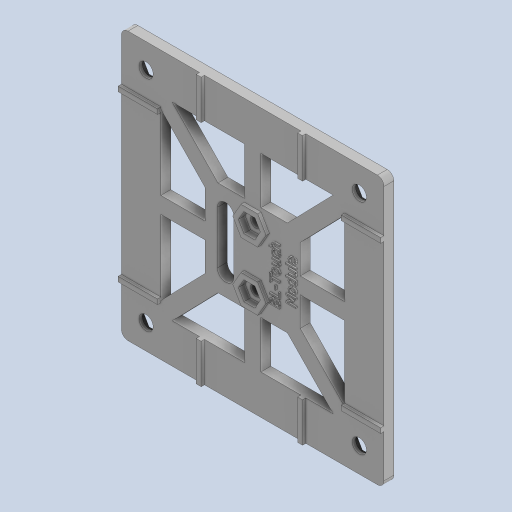
# Autodesk Inventor part: BLTouch-LevelingPlate
Saved by Autodesk Inventor 2023.2 (Build 272271000, 271)
## iProperties
Created: 2024-02-15
Part Number: BLTouch-LevelingPlate
Material: Generisch
Document SubType Name: Modeling
Designer: Nils Bade
Density: 1 g/cm^3
Appearance: PLA Druck IHF
Description: Dummy
Auf Bestellliste: True
Author: Nils Bade
Autodesk Inventor part; units mm, degrees
ref_plane "YZ Plane" through (0, 0, 0) normal (1, 0, 0) x (0, 1, 0)
ref_plane "XZ Plane" through (0, 0, 0) normal (0, 1, 0) x (-1, 0, 0)
ref_plane "XY Plane" through (0, 0, 0) normal (0, 0, 1) x (1, 0, 0)
sketch "S-Basis" plane through (0, 0, 0) normal (0, 0, 1) x (1, 0, 0)
  line L0 (0, 57.19) -> (0, -57.19) construction
  line L1 (-56, 0) -> (56, 0) construction
  line L2 (-40, 40.85) -> (40, 40.85)
  line L3 (40, 40.85) -> (40, -40.85)
  line L4 (40, -40.85) -> (-40, -40.85)
  line L5 (-40, -40.85) -> (-40, 40.85)
  line L6 (-40, 40.85) -> (40, -40.85) construction
  line L7 (40, 40.85) -> (-40, -40.85) construction
  line L8 (-40, 33.35) -> (40, 33.35) construction
  circle A0 centre (0, 33.35) radius 2.5 construction
  circle A1 centre (-32.5, 33.35) radius 2.15
  circle A2 centre (32.5, 33.35) radius 2.15
  circle A3 centre (-32.5, -33.35) radius 2.15
  circle A4 centre (32.5, -33.35) radius 2.15
  line L9 (-3.5, 40.85) -> (3.5, 40.85)
  line L10 (7.5, 31.85) -> (5, 31.85)
  line L11 (5, 31.85) -> (5, 37.85)
  line L12 (5, 37.85) -> (7.5, 37.85)
  line L13 (7.5, 37.85) -> (7.5, 31.85)
  line L14 (-7.5, 31.85) -> (-5, 31.85)
  line L15 (-5, 31.85) -> (-5, 37.85)
  line L16 (-5, 37.85) -> (-7.5, 37.85)
  line L17 (-7.5, 37.85) -> (-7.5, 31.85)
  point P0 (0, 40.85)
  point P1 (0, 0)
  point P2 (0, 0)
  dimension "d0" = 81.7
  dimension "d1" = 80
  dimension "d4" = 7.5
  dimension "d7" = 4.3
  dimension "d8" = 32.5
  dimension "d9" = 4.3
  dimension "d10" = 32.5
  dimension "d11" = 7.5
  dimension "d60" = 6
  dimension "d61" = 2.5
  dimension "d62" = 5
  dimension "d63" = 3
  constraints: 32 end point, 6 midpoint, 6 symmetric about line, 5 centre point, 5 point on line, 4 parallel, 3 horizontal, 3 perpendicular, 2 other
  measures "d0" distance of L2.end L3.end
  measures "d1" distance of L2.start L2.end
  measures "d4" distance between parallel lines of L8 L2
  measures "d7" diameter of A1
  measures "d8" distance from line of L0 A1.centre
  measures "d9" diameter of A3
  measures "d10" distance from line of L0 A3.centre
  measures "d11" distance from line of L4 A3.centre
  measures "d60" distance of L12.end L10.start
  measures "d61" distance between parallel lines of L13 L11
  measures "d62" distance between parallel lines of L0 L11
  measures "d63" distance between parallel lines of L12 L2
extrude "Ex-Base1" add sketch "S-Basis" against normal blind 3 contours L2 L3 L4 L5 | L10 L11 L12 L13 | L17 L16 L15 L14
fillet "Rundung-2mm" radius 2 4 edges at (40, -40.85, -1.5) (-40, -40.85, -1.5) (40, 40.85, -1.5) (-40, 40.85, -1.5)
sketch "S-BLTouch-Mount" plane through (0, 0, 0) normal (0, 0, 1) x (1, 0, 0)
  line L0 (0, 9) -> (0, -9) construction
  line L1 (-4.4389, 9) -> (-4.4389, -9) construction
  line L2 (4.4389, -9) -> (4.4389, 9) construction
  arc A0 (4.4389, 9) -> (-4.4389, 9) centre (0, 9) ccw construction
  arc A1 (-4.4389, -9) -> (4.4389, -9) centre (0, -9) ccw construction
  circle A2 centre (0, -9) radius 1.65
  line L3 (0, 57.19) -> (0, -57.19) construction
  line L4 (-56, 0) -> (56, 0) construction
  line L5 (-1.6743, -6.1) -> (1.6743, -6.1)
  line L6 (1.6743, -6.1) -> (3.3486, -9)
  line L7 (3.3486, -9) -> (1.6743, -11.9)
  line L8 (1.6743, -11.9) -> (-1.6743, -11.9)
  line L9 (-1.6743, -11.9) -> (-3.3486, -9)
  line L10 (-3.3486, -9) -> (-1.6743, -6.1)
  circle A3 centre (0, 0) radius 3
  line L11 (-8.25, 8) -> (-8.25, -8) construction
  line L12 (-10.75, 8) -> (-10.75, -8)
  line L13 (-5.75, -8) -> (-5.75, 8)
  arc A4 (-5.75, 8) -> (-10.75, 8) centre (-8.25, 8) ccw
  arc A5 (-10.75, -8) -> (-5.75, -8) centre (-8.25, -8) ccw
  circle A6 centre (0, 9) radius 1.65
  line L14 (-1.6743, 6.1) -> (1.6743, 6.1)
  line L15 (1.6743, 6.1) -> (3.3486, 9)
  line L16 (3.3486, 9) -> (1.6743, 11.9)
  line L17 (1.6743, 11.9) -> (-1.6743, 11.9)
  line L18 (-1.6743, 11.9) -> (-3.3486, 9)
  line L19 (-3.3486, 9) -> (-1.6743, 6.1)
  line L20 (-5.0807, -9) -> (-2.5403, -13.4)
  line L21 (-2.5403, -13.4) -> (2.5403, -13.4)
  line L22 (2.5403, -13.4) -> (5.0807, -9)
  line L23 (5.0807, -9) -> (2.5403, -4.6)
  line L24 (2.5403, -4.6) -> (-2.5403, -4.6)
  line L25 (-2.5403, -4.6) -> (-5.0807, -9)
  line L26 (-2.5403, 4.6) -> (2.5403, 4.6)
  line L27 (2.5403, 4.6) -> (5.0807, 9)
  line L28 (5.0807, 9) -> (2.5403, 13.4)
  line L29 (2.5403, 13.4) -> (-2.5403, 13.4)
  line L30 (-2.5403, 13.4) -> (-5.0807, 9)
  line L31 (-5.0807, 9) -> (-2.5403, 4.6)
  line L32 (-14.5, -14.5) -> (14.5, -14.5)
  line L33 (14.5, -14.5) -> (14.5, 14.5)
  line L34 (14.5, 14.5) -> (-14.5, 14.5)
  line L35 (-14.5, 14.5) -> (-14.5, -14.5)
  line L36 (-14.5, -14.5) -> (14.5, 14.5) construction
  line L37 (14.5, -14.5) -> (-14.5, 14.5) construction
  line L38 (28, -28.85) -> (-28, -28.85)
  line L39 (-28, -28.85) -> (-28, 28.85)
  line L40 (-28, 28.85) -> (28, 28.85)
  line L41 (28, 28.85) -> (28, -28.85)
  line L42 (28, -28.85) -> (-28, 28.85) construction
  line L43 (-28, -28.85) -> (28, 28.85) construction
  line L44 (40, -38.85) -> (40, 38.85) projected
  line L45 (-40, 38.85) -> (-40, -38.85) projected
  line L46 (-38, -40.85) -> (38, -40.85) projected
  line L47 (2.5, -28.85) -> (2.5, -14.5)
  line L48 (10.589, -14.5) -> (24.5162, -28.85)
  line L49 (14.5, -11.3506) -> (28, -25.2604)
  line L50 (14.5, -2.5) -> (28, -2.5)
  line L51 (2.5, 28.85) -> (2.5, 14.5)
  line L52 (10.589, 14.5) -> (24.5162, 28.85)
  line L53 (14.5, 11.3506) -> (28, 25.2604)
  line L54 (14.5, 2.5) -> (28, 2.5)
  line L55 (-2.5, -28.85) -> (-2.5, -14.5)
  line L56 (-10.589, -14.5) -> (-24.5162, -28.85)
  line L57 (-14.5, -11.3506) -> (-28, -25.2604)
  line L58 (-14.5, -2.5) -> (-28, -2.5)
  line L59 (-2.5, 28.85) -> (-2.5, 14.5)
  line L60 (-10.589, 14.5) -> (-24.5162, 28.85)
  line L61 (-14.5, 11.3506) -> (-28, 25.2604)
  line L62 (-14.5, 2.5) -> (-28, 2.5)
  line L63 (5.3885, -14.3851) -> (5.3885, 14.3851) construction
  line L64 (5.3885, 14.3851) -> (13.9659, 14.3851) construction
  line L65 (13.9659, 14.3851) -> (13.9659, -14.3851) construction
  line L66 (13.9659, -14.3851) -> (5.3885, -14.3851) construction
  spline S0 degree 2 poles (7.6363, -6.9815) (7.8635, -6.9815) (8.2118, -7.1544) (8.3254, -7.2977) knots 0 0 0 1 2 2 2
  spline S1 degree 2 poles (8.3254, -7.2977) (8.4588, -7.4706) (8.5724, -7.8633) (8.5724, -8.1745) knots 0 0 0 1 2 2 2
  line L67 (8.5724, -8.1745) -> (8.5724, -9.0489)
  line L68 (8.5724, -9.0489) -> (5.5244, -9.0489)
  line L69 (5.5244, -9.0489) -> (5.5244, -8.2412)
  spline S2 degree 2 poles (5.5244, -8.2412) (5.5244, -7.9152) (5.5664, -7.5891) (5.6479, -7.4409) knots 0 0 0 1 2 2 2
  spline S3 degree 2 poles (5.6479, -7.4409) (5.7343, -7.2754) (6.0184, -7.1248) (6.2111, -7.1248) knots 0 0 0 1 2 2 2
  spline S4 degree 2 poles (6.2111, -7.1248) (6.4259, -7.1248) (6.7668, -7.352) (6.8631, -7.5521) knots 0 0 0 1 2 2 2
  line L70 (6.8631, -7.5521) -> (6.878, -7.5521)
  spline S5 degree 2 poles (6.878, -7.5521) (6.9521, -7.2804) (7.3448, -6.9815) (7.6363, -6.9815) knots 0 0 0 1 2 2 2
  spline S6 degree 2 poles (7.6535, -7.4039) (7.4806, -7.4039) (7.2583, -7.5027) (7.1793, -7.6509) knots 0 0 0 1 2 2 2
  spline S7 degree 2 poles (7.1793, -7.6509) (7.1299, -7.7472) (7.1003, -7.9744) (7.1003, -8.1844) knots 0 0 0 1 2 2 2
  line L71 (7.1003, -8.1844) -> (7.1003, -8.6438)
  line L72 (7.1003, -8.6438) -> (8.2266, -8.6438)
  line L73 (8.2266, -8.6438) -> (8.2266, -8.3153)
  spline S8 degree 2 poles (8.2266, -8.3153) (8.2266, -8.0485) (8.1772, -7.7423) (8.0981, -7.6237) knots 0 0 0 1 2 2 2
  spline S9 degree 2 poles (8.0981, -7.6237) (8.0166, -7.5101) (7.8141, -7.4039) (7.6535, -7.4039) knots 0 0 0 1 2 2 2
  spline S10 degree 2 poles (6.2679, -7.5471) (6.1592, -7.5471) (5.9962, -7.6212) (5.9492, -7.7027) knots 0 0 0 1 2 2 2
  spline S11 degree 2 poles (5.9492, -7.7027) (5.8949, -7.8015) (5.8702, -8.0411) (5.8702, -8.256) knots 0 0 0 1 2 2 2
  line L74 (5.8702, -8.256) -> (5.8702, -8.6438)
  line L75 (5.8702, -8.6438) -> (6.7619, -8.6438)
  line L76 (6.7619, -8.6438) -> (6.7619, -8.1844)
  spline S12 degree 2 poles (6.7619, -8.1844) (6.7619, -7.9942) (6.7223, -7.8139) (6.6606, -7.7176) knots 0 0 0 1 2 2 2
  spline S13 degree 2 poles (6.6606, -7.7176) (6.6013, -7.6237) (6.4111, -7.5471) (6.2679, -7.5471) knots 0 0 0 1 2 2 2
  line L77 (8.5724, -4.8128) -> (8.5724, -6.5789)
  line L78 (8.5724, -6.5789) -> (5.5244, -6.5789)
  line L79 (5.5244, -6.5789) -> (5.5244, -6.1738)
  line L80 (5.5244, -6.1738) -> (8.2118, -6.1738)
  line L81 (8.2118, -6.1738) -> (8.2118, -4.8128)
  line L82 (8.2118, -4.8128) -> (8.5724, -4.8128)
  line L83 (7.4238, -3.4642) -> (7.4238, -4.6177)
  line L84 (7.4238, -4.6177) -> (7.0533, -4.6177)
  line L85 (7.0533, -4.6177) -> (7.0533, -3.4642)
  line L86 (7.0533, -3.4642) -> (7.4238, -3.4642)
  line L87 (8.5724, -2.2613) -> (5.885, -2.2613)
  line L88 (5.885, -2.2613) -> (5.885, -3.2839)
  line L89 (5.885, -3.2839) -> (5.5244, -3.2839)
  line L90 (5.5244, -3.2839) -> (5.5244, -0.8336)
  line L91 (5.5244, -0.8336) -> (5.885, -0.8336)
  line L92 (5.885, -0.8336) -> (5.885, -1.8562)
  line L93 (5.885, -1.8562) -> (8.5724, -1.8562)
  line L94 (8.5724, -1.8562) -> (8.5724, -2.2613)
  spline S14 degree 2 poles (7.4288, 1.3252) (8.0068, 1.3252) (8.6366, 0.7694) (8.6366, 0.305) knots 0 0 0 1 2 2 2
  spline S15 degree 2 poles (8.6366, 0.305) (8.6366, -0.1717) (7.987, -0.7175) (7.4288, -0.7175) knots 0 0 0 1 2 2 2
  spline S16 degree 2 poles (7.4288, -0.7175) (6.8557, -0.7175) (6.2209, -0.1544) (6.2209, 0.305) knots 0 0 0 1 2 2 2
  spline S17 degree 2 poles (6.2209, 0.305) (6.2209, 0.7694) (6.8533, 1.3252) (7.4288, 1.3252) knots 0 0 0 1 2 2 2
  spline S18 degree 2 poles (7.4288, 0.9275) (6.9842, 0.9275) (6.5519, 0.6039) (6.5519, 0.305) knots 0 0 0 1 2 2 2
  spline S19 degree 2 poles (6.5519, 0.305) (6.5519, 0.0062) (6.9842, -0.3199) (7.4288, -0.3199) knots 0 0 0 1 2 2 2
  spline S20 degree 2 poles (7.4288, -0.3199) (7.861, -0.3199) (8.3056, 0.0062) (8.3056, 0.305) knots 0 0 0 1 2 2 2
  spline S21 degree 2 poles (8.3056, 0.305) (8.3056, 0.6014) (7.8684, 0.9275) (7.4288, 0.9275) knots 0 0 0 1 2 2 2
  line L95 (8.5724, 3.4988) -> (8.5724, 3.1135)
  line L96 (8.5724, 3.1135) -> (8.3204, 3.1135)
  spline S22 degree 2 poles (8.3204, 3.1135) (8.4761, 2.9356) (8.6366, 2.617) (8.6366, 2.4194) knots 0 0 0 1 2 2 2
  spline S23 degree 2 poles (8.6366, 2.4194) (8.6366, 2.2712) (8.5378, 2.0069) (8.4316, 1.9106) knots 0 0 0 1 2 2 2
  spline S24 degree 2 poles (8.4316, 1.9106) (8.3254, 1.8118) (8.0018, 1.7031) (7.7696, 1.7031) knots 0 0 0 1 2 2 2
  line L97 (7.7696, 1.7031) -> (6.2852, 1.7031)
  line L98 (6.2852, 1.7031) -> (6.2852, 2.0884)
  line L99 (6.2852, 2.0884) -> (7.5893, 2.0884)
  spline S25 degree 2 poles (7.5893, 2.0884) (7.7721, 2.0884) (8.0117, 2.1156) (8.1006, 2.1625) knots 0 0 0 1 2 2 2
  spline S26 degree 2 poles (8.1006, 2.1625) (8.1895, 2.2094) (8.271, 2.37) (8.271, 2.5207) knots 0 0 0 1 2 2 2
  spline S27 degree 2 poles (8.271, 2.5207) (8.271, 2.6614) (8.1105, 2.9801) (7.9944, 3.1135) knots 0 0 0 1 2 2 2
  line L100 (7.9944, 3.1135) -> (6.2852, 3.1135)
  line L101 (6.2852, 3.1135) -> (6.2852, 3.4988)
  line L102 (6.2852, 3.4988) -> (8.5724, 3.4988)
  spline S28 degree 2 poles (8.6243, 4.966) (8.6243, 4.7288) (8.4785, 4.3361) (8.3303, 4.1953) knots 0 0 0 1 2 2 2
  spline S29 degree 2 poles (8.3303, 4.1953) (8.1846, 4.0545) (7.7351, 3.8989) (7.4337, 3.8989) knots 0 0 0 1 2 2 2
  spline S30 degree 2 poles (7.4337, 3.8989) (7.1324, 3.8989) (6.6927, 4.0595) (6.5445, 4.1953) knots 0 0 0 1 2 2 2
  spline S31 degree 2 poles (6.5445, 4.1953) (6.3938, 4.3312) (6.2333, 4.7338) (6.2333, 4.966) knots 0 0 0 1 2 2 2
  spline S32 degree 2 poles (6.2333, 4.966) (6.2333, 5.1537) (6.3395, 5.5044) (6.4087, 5.6403) knots 0 0 0 1 2 2 2
  line L103 (6.4087, 5.6403) -> (6.8409, 5.6403)
  line L104 (6.8409, 5.6403) -> (6.8409, 5.6181)
  spline S33 degree 2 poles (6.8409, 5.6181) (6.8063, 5.5761) (6.7174, 5.4476) (6.6705, 5.3562) knots 0 0 0 1 2 2 2
  spline S34 degree 2 poles (6.6705, 5.3562) (6.631, 5.2747) (6.5692, 5.0574) (6.5692, 4.9586) knots 0 0 0 1 2 2 2
  spline S35 degree 2 poles (6.5692, 4.9586) (6.5692, 4.6597) (7.0212, 4.2966) (7.4337, 4.2966) knots 0 0 0 1 2 2 2
  spline S36 degree 2 poles (7.4337, 4.2966) (7.8363, 4.2966) (8.2883, 4.6473) (8.2883, 4.9586) knots 0 0 0 1 2 2 2
  spline S37 degree 2 poles (8.2883, 4.9586) (8.2883, 5.1463) (8.1327, 5.4871) (8.0117, 5.6181) knots 0 0 0 1 2 2 2
  line L105 (8.0117, 5.6181) -> (8.0117, 5.6403)
  line L106 (8.0117, 5.6403) -> (8.4439, 5.6403)
  spline S38 degree 2 poles (8.4439, 5.6403) (8.4711, 5.5835) (8.5477, 5.4106) (8.565, 5.3414) knots 0 0 0 1 2 2 2
  spline S39 degree 2 poles (8.565, 5.3414) (8.5946, 5.2426) (8.6243, 5.087) (8.6243, 4.966) knots 0 0 0 1 2 2 2
  line L107 (8.5724, 7.7867) -> (8.5724, 7.4014)
  line L108 (8.5724, 7.4014) -> (7.2682, 7.4014)
  spline S40 degree 2 poles (7.2682, 7.4014) (7.1101, 7.4014) (6.8384, 7.3718) (6.7569, 7.3273) knots 0 0 0 1 2 2 2
  spline S41 degree 2 poles (6.7569, 7.3273) (6.6705, 7.2804) (6.5865, 7.1124) (6.5865, 6.9692) knots 0 0 0 1 2 2 2
  spline S42 degree 2 poles (6.5865, 6.9692) (6.5865, 6.8259) (6.7396, 6.5221) (6.8631, 6.3763) knots 0 0 0 1 2 2 2
  line L109 (6.8631, 6.3763) -> (8.5724, 6.3763)
  line L110 (8.5724, 6.3763) -> (8.5724, 5.991)
  line L111 (8.5724, 5.991) -> (5.3885, 5.991)
  line L112 (5.3885, 5.991) -> (5.3885, 6.3763)
  line L113 (5.3885, 6.3763) -> (6.5396, 6.3763)
  spline S43 degree 2 poles (6.5396, 6.3763) (6.384, 6.5492) (6.2209, 6.8827) (6.2209, 7.0704) knots 0 0 0 1 2 2 2
  spline S44 degree 2 poles (6.2209, 7.0704) (6.2209, 7.4063) (6.6655, 7.7867) (7.0879, 7.7867) knots 0 0 0 1 2 2 2
  line L114 (7.0879, 7.7867) -> (8.5724, 7.7867)
  line L115 (13.5908, -3.7396) -> (13.5908, -4.1447)
  line L116 (13.5908, -4.1447) -> (10.9652, -4.1447)
  line L117 (10.9652, -4.1447) -> (12.751, -4.94)
  line L118 (12.751, -4.94) -> (12.751, -5.187)
  line L119 (12.751, -5.187) -> (10.9652, -5.975)
  line L120 (10.9652, -5.975) -> (13.5908, -5.975)
  line L121 (13.5908, -5.975) -> (13.5908, -6.3529)
  line L122 (13.5908, -6.3529) -> (10.5428, -6.3529)
  line L123 (10.5428, -6.3529) -> (10.5428, -5.7996)
  line L124 (10.5428, -5.7996) -> (12.2397, -5.0388)
  line L125 (12.2397, -5.0388) -> (10.5428, -4.3028)
  line L126 (10.5428, -4.3028) -> (10.5428, -3.7396)
  line L127 (10.5428, -3.7396) -> (13.5908, -3.7396)
  spline S45 degree 2 poles (12.4472, -1.2721) (13.0252, -1.2721) (13.6551, -1.8278) (13.6551, -2.2922) knots 0 0 0 1 2 2 2
  spline S46 degree 2 poles (13.6551, -2.2922) (13.6551, -2.7689) (13.0054, -3.3148) (12.4472, -3.3148) knots 0 0 0 1 2 2 2
  spline S47 degree 2 poles (12.4472, -3.3148) (11.8742, -3.3148) (11.2394, -2.7516) (11.2394, -2.2922) knots 0 0 0 1 2 2 2
  spline S48 degree 2 poles (11.2394, -2.2922) (11.2394, -1.8278) (11.8717, -1.2721) (12.4472, -1.2721) knots 0 0 0 1 2 2 2
  spline S49 degree 2 poles (12.4472, -1.6697) (12.0026, -1.6697) (11.5704, -1.9933) (11.5704, -2.2922) knots 0 0 0 1 2 2 2
  spline S50 degree 2 poles (11.5704, -2.2922) (11.5704, -2.591) (12.0026, -2.9171) (12.4472, -2.9171) knots 0 0 0 1 2 2 2
  spline S51 degree 2 poles (12.4472, -2.9171) (12.8795, -2.9171) (13.3241, -2.591) (13.3241, -2.2922) knots 0 0 0 1 2 2 2
  spline S52 degree 2 poles (13.3241, -2.2922) (13.3241, -1.9958) (12.8869, -1.6697) (12.4472, -1.6697) knots 0 0 0 1 2 2 2
  line L128 (13.5908, 0.8818) -> (13.5908, 0.4965)
  line L129 (13.5908, 0.4965) -> (13.3587, 0.4965)
  spline S53 degree 2 poles (13.3587, 0.4965) (13.4328, 0.4076) (13.5316, 0.2766) (13.5735, 0.1877) knots 0 0 0 1 2 2 2
  spline S54 degree 2 poles (13.5735, 0.1877) (13.6131, 0.1062) (13.6551, -0.0692) (13.6551, -0.1853) knots 0 0 0 1 2 2 2
  spline S55 degree 2 poles (13.6551, -0.1853) (13.6551, -0.373) (13.4994, -0.6891) (13.3488, -0.8003) knots 0 0 0 1 2 2 2
  spline S56 degree 2 poles (13.3488, -0.8003) (13.1981, -0.9114) (12.7535, -1.0349) (12.4645, -1.0349) knots 0 0 0 1 2 2 2
  spline S57 degree 2 poles (12.4645, -1.0349) (12.1632, -1.0349) (11.7235, -0.8793) (11.558, -0.7435) knots 0 0 0 1 2 2 2
  spline S58 degree 2 poles (11.558, -0.7435) (11.4098, -0.6175) (11.2394, -0.2643) (11.2394, -0.0692) knots 0 0 0 1 2 2 2
  spline S59 degree 2 poles (11.2394, -0.0692) (11.2394, 0.1013) (11.316, 0.3557) (11.395, 0.4965) knots 0 0 0 1 2 2 2
  line L130 (11.395, 0.4965) -> (10.407, 0.4965)
  line L131 (10.407, 0.4965) -> (10.407, 0.8818)
  line L132 (10.407, 0.8818) -> (13.5908, 0.8818)
  line L133 (13.0351, 0.4965) -> (11.7136, 0.4965)
  spline S60 degree 2 poles (11.7136, 0.4965) (11.6445, 0.3532) (11.5926, 0.126) (11.5926, -0.0049) knots 0 0 0 1 2 2 2
  spline S61 degree 2 poles (11.5926, -0.0049) (11.5926, -0.3013) (12.0372, -0.6373) (12.4571, -0.6373) knots 0 0 0 1 2 2 2
  spline S62 degree 2 poles (12.4571, -0.6373) (12.8622, -0.6373) (13.2895, -0.3804) (13.2895, -0.0963) knots 0 0 0 1 2 2 2
  spline S63 degree 2 poles (13.2895, -0.0963) (13.2895, 0.0543) (13.1512, 0.3606) (13.0351, 0.4965) knots 0 0 0 1 2 2 2
  line L134 (13.5908, 3.2184) -> (13.5908, 2.8331)
  line L135 (13.5908, 2.8331) -> (13.3389, 2.8331)
  spline S64 degree 2 poles (13.3389, 2.8331) (13.4945, 2.6553) (13.6551, 2.3366) (13.6551, 2.139) knots 0 0 0 1 2 2 2
  spline S65 degree 2 poles (13.6551, 2.139) (13.6551, 1.9908) (13.5563, 1.7265) (13.45, 1.6302) knots 0 0 0 1 2 2 2
  spline S66 degree 2 poles (13.45, 1.6302) (13.3438, 1.5314) (13.0203, 1.4227) (12.7881, 1.4227) knots 0 0 0 1 2 2 2
  line L136 (12.7881, 1.4227) -> (11.3036, 1.4227)
  line L137 (11.3036, 1.4227) -> (11.3036, 1.8081)
  line L138 (11.3036, 1.8081) -> (12.6078, 1.8081)
  spline S67 degree 2 poles (12.6078, 1.8081) (12.7906, 1.8081) (13.0301, 1.8352) (13.1191, 1.8822) knots 0 0 0 1 2 2 2
  spline S68 degree 2 poles (13.1191, 1.8822) (13.208, 1.9291) (13.2895, 2.0896) (13.2895, 2.2403) knots 0 0 0 1 2 2 2
  spline S69 degree 2 poles (13.2895, 2.2403) (13.2895, 2.3811) (13.1289, 2.6997) (13.0129, 2.8331) knots 0 0 0 1 2 2 2
  line L139 (13.0129, 2.8331) -> (11.3036, 2.8331)
  line L140 (11.3036, 2.8331) -> (11.3036, 3.2184)
  line L141 (11.3036, 3.2184) -> (13.5908, 3.2184)
  line L142 (13.5908, 4.1694) -> (13.5908, 3.7841)
  line L143 (13.5908, 3.7841) -> (10.407, 3.7841)
  line L144 (10.407, 3.7841) -> (10.407, 4.1694)
  line L145 (10.407, 4.1694) -> (13.5908, 4.1694)
  spline S70 degree 2 poles (13.6427, 5.728) (13.6427, 5.1796) (13.0277, 4.5769) (12.4596, 4.5769) knots 0 0 0 1 2 2 2
  spline S71 degree 2 poles (12.4596, 4.5769) (11.9013, 4.5769) (11.2394, 5.1623) (11.2394, 5.6341) knots 0 0 0 1 2 2 2
  spline S72 degree 2 poles (11.2394, 5.6341) (11.2394, 5.8465) (11.3629, 6.175) (11.4938, 6.2961) knots 0 0 0 1 2 2 2
  spline S73 degree 2 poles (11.4938, 6.2961) (11.6247, 6.4196) (12.0026, 6.5505) (12.2768, 6.5505) knots 0 0 0 1 2 2 2
  line L146 (12.2768, 6.5505) -> (12.4867, 6.5505)
  line L147 (12.4867, 6.5505) -> (12.4867, 4.9672)
  spline S74 degree 2 poles (12.4867, 4.9672) (12.8844, 4.9672) (13.3068, 5.3673) (13.3068, 5.723) knots 0 0 0 1 2 2 2
  spline S75 degree 2 poles (13.3068, 5.723) (13.3068, 5.849) (13.25, 6.0935) (13.2055, 6.1923) knots 0 0 0 1 2 2 2
  spline S76 degree 2 poles (13.2055, 6.1923) (13.1561, 6.2961) (13.0697, 6.4393) (13.0301, 6.4863) knots 0 0 0 1 2 2 2
  line L148 (13.0301, 6.4863) -> (13.0301, 6.5085)
  line L149 (13.0301, 6.5085) -> (13.45, 6.5085)
  spline S77 degree 2 poles (13.45, 6.5085) (13.4772, 6.4418) (13.5563, 6.2393) (13.5785, 6.1602) knots 0 0 0 1 2 2 2
  spline S78 degree 2 poles (13.5785, 6.1602) (13.6106, 6.0491) (13.6427, 5.8663) (13.6427, 5.728) knots 0 0 0 1 2 2 2
  spline S79 degree 2 poles (12.1928, 6.175) (12.0372, 6.1701) (11.81, 6.1059) (11.7334, 6.0441) knots 0 0 0 1 2 2 2
  spline S80 degree 2 poles (11.7334, 6.0441) (11.6469, 5.9774) (11.5555, 5.7675) (11.5555, 5.6119) knots 0 0 0 1 2 2 2
  spline S81 degree 2 poles (11.5555, 5.6119) (11.5555, 5.4587) (11.6469, 5.2438) (11.7359, 5.1549) knots 0 0 0 1 2 2 2
  spline S82 degree 2 poles (11.7359, 5.1549) (11.8272, 5.0685) (12.0471, 4.9796) (12.1928, 4.9672) knots 0 0 0 1 2 2 2
  line L150 (12.1928, 4.9672) -> (12.1928, 6.175)
  point P0 (-8.25, 0)
  point P1 (5.3885, 0)
  dimension "d26" = 18
  dimension "d27" = 3.3
  dimension "d28" = 5.8
  dimension "d29" = 6
  dimension "d30" = 5.75
  dimension "d31" = 5
  dimension "d32" = 16
  dimension "d39" = 1.5
  dimension "d40" = 1.5
  dimension "d43" = 29
  dimension "d44" = 29
  dimension "d45" = 12
  dimension "d46" = 12
  dimension "d47" = 2.5
  dimension "d48" = 5
  dimension "d49" = 2.5
  constraints: 120 end point, 32 symmetric about line, 10 point on line, 8 point on circle, 8 tangent, 7 centre point, 7 midpoint, 7 parallel, 5 coincident, 5 perpendicular, 3 horizontal, 1 vertical, 27 other
  measures "d26" distance of L0.start L0.end
  measures "d27" diameter of A2
  measures "d28" distance between parallel lines of L8 L5
  measures "d29" diameter of A3
  measures "d30" distance between parallel lines of L13 L3
  measures "d31" distance between parallel lines of L13 L12
  measures "d32" distance of L12.start L12.end
  measures "d39" distance between parallel lines of L9 L20
  measures "d40" distance between parallel lines of L19 L31
  measures "d43" distance of L34.end L33.end
  measures "d44" distance of L33.end L32.end
  measures "d45" distance between parallel lines of L38 L46
  measures "d46" distance between parallel lines of L45 L39
  measures "d47" distance between parallel lines of L4 L50
  measures "d48" distance between parallel lines of L49 L48
  measures "d49" distance between parallel lines of L3 L47
extrude "Ex-BLTouch-Mount1" cut sketch "S-BLTouch-Mount" against normal blind 10 contours A2 | A4 L13 A5 L12 | A6
extrude "Ex-BLTouch-Mount2" cut sketch "S-BLTouch-Mount" along normal blind 1 from surface at -3 contours A3
extrude "Ex-BLTouch-Mount3" cut sketch "S-BLTouch-Mount" against normal blind 1 contours L5 L6 L7 L8 L9 L10 | L19 L18 L17 L16 L15 L14
extrude "Ex-BLTouch-Mount4" add sketch "S-BLTouch-Mount" along normal blind 1 contours L25 L24 L23 L22 L21 L20 | L31 L30 L29 L28 L27 L26
extrude "Ex-LightWeightBABY" cut sketch "S-BLTouch-Mount" against normal blind 3 contours L32 L55 L38 L56 | L57 L39 L58 L35 | L32 L48 L38 L47 | L62 L39 L61 L35 | L33 L50 L41 L49 | L60 L40 L59 L34 | L33 L53 L41 L54 | L51 L40 L52 L34
extrude "Ex-Beschriftung" add sketch "S-BLTouch-Mount" along normal blind 0.5 contours S0 S1 L67 L68 L69 S2 S3 S4 L70 S5 | L77 L78 L79 L80 L81 L82 | L83 L84 L85 L86 | L87 L88 L89 L90 L91 L92 L93 L94 | S14 S15 S16 S17 | L95 L96 S22 S23 S24 L97 L98 L99 S25 S26 S27 L100 L101 L102 | S28 S29 S30 S31 S32 L103 L104 S33 S34 S35 S36 S37 L105 L106 S38 S39 | L107 L108 S40 S41 S42 L109 L110 L111 L112 L113 S43 S44 L114 | L115 L116 L117 L118 L119 L120 L121 L122 L123 L124 L125 L126 L127 | S45 S46 S47 S48 | L128 L129 S53 S54 S55 S56 S57 S58 S59 L130 L131 L132 | L134 L135 S64 S65 S66 L136 L137 L138 S67 S68 S69 L139 L140 L141 | L142 L143 L144 L145 | S70 S71 S72 S73 L146 L147 S74 S75 S76 L148 L149 S77 S78
sketch "S-PlateMount" plane through (0, 0, 0) normal (0, 0, 1) x (1, 0, 0)
  circle A0 centre (32.5, -33.35) radius 2.15 projected
  line L0 (-53.8254, 0) -> (53.8254, 0) construction
  line L1 (0, 53.9) -> (0, -53.9) construction
  circle A1 centre (32.5, -33.35) radius 2.15 projected
  line L2 (30.3927, -29.7) -> (34.6073, -29.7)
  line L3 (34.6073, -29.7) -> (36.7147, -33.35)
  line L4 (36.7147, -33.35) -> (34.6073, -37)
  line L5 (34.6073, -37) -> (30.3927, -37)
  line L6 (30.3927, -37) -> (28.2853, -33.35)
  line L7 (28.2853, -33.35) -> (30.3927, -29.7)
  line L8 (26.5533, -33.35) -> (29.5266, -38.5)
  line L9 (29.5266, -38.5) -> (35.4734, -38.5)
  line L10 (35.4734, -38.5) -> (38.4467, -33.35)
  line L11 (38.4467, -33.35) -> (35.4734, -28.2)
  line L12 (35.4734, -28.2) -> (29.5266, -28.2)
  line L13 (29.5266, -28.2) -> (26.5533, -33.35)
  line L14 (-30.3927, -29.7) -> (-34.6073, -29.7)
  line L15 (-34.6073, -29.7) -> (-36.7147, -33.35)
  line L16 (-36.7147, -33.35) -> (-34.6073, -37)
  line L17 (-34.6073, -37) -> (-30.3927, -37)
  line L18 (-30.3927, -37) -> (-28.2853, -33.35)
  line L19 (-28.2853, -33.35) -> (-30.3927, -29.7)
  line L20 (-26.5533, -33.35) -> (-29.5266, -38.5)
  line L21 (-29.5266, -38.5) -> (-35.4734, -38.5)
  line L22 (-35.4734, -38.5) -> (-38.4467, -33.35)
  line L23 (-38.4467, -33.35) -> (-35.4734, -28.2)
  line L24 (-35.4734, -28.2) -> (-29.5266, -28.2)
  line L25 (-29.5266, -28.2) -> (-26.5533, -33.35)
  line L26 (30.3927, 29.7) -> (34.6073, 29.7)
  line L27 (34.6073, 29.7) -> (36.7147, 33.35)
  line L28 (36.7147, 33.35) -> (34.6073, 37)
  line L29 (34.6073, 37) -> (30.3927, 37)
  line L30 (30.3927, 37) -> (28.2853, 33.35)
  line L31 (28.2853, 33.35) -> (30.3927, 29.7)
  line L32 (26.5533, 33.35) -> (29.5266, 38.5)
  line L33 (29.5266, 38.5) -> (35.4734, 38.5)
  line L34 (35.4734, 38.5) -> (38.4467, 33.35)
  line L35 (38.4467, 33.35) -> (35.4734, 28.2)
  line L36 (35.4734, 28.2) -> (29.5266, 28.2)
  line L37 (29.5266, 28.2) -> (26.5533, 33.35)
  line L38 (-26.5533, 33.35) -> (-29.5266, 38.5)
  line L39 (-30.3927, 37) -> (-28.2853, 33.35)
  line L40 (-34.6073, 37) -> (-30.3927, 37)
  line L41 (-29.5266, 38.5) -> (-35.4734, 38.5)
  line L42 (-28.2853, 33.35) -> (-30.3927, 29.7)
  line L43 (-29.5266, 28.2) -> (-26.5533, 33.35)
  line L44 (-36.7147, 33.35) -> (-34.6073, 37)
  line L45 (-30.3927, 29.7) -> (-34.6073, 29.7)
  line L46 (-35.4734, 28.2) -> (-29.5266, 28.2)
  line L47 (-34.6073, 29.7) -> (-36.7147, 33.35)
  line L48 (-38.4467, 33.35) -> (-35.4734, 28.2)
  line L49 (-35.4734, 38.5) -> (-38.4467, 33.35)
  line L50 (16.2, -40.85) -> (16.2, -28.85)
  line L51 (40, -38.85) -> (40, 38.85) projected
  line L52 (-38, -40.85) -> (38, -40.85) projected
  line L53 (24.5162, -28.85) -> (2.5, -28.85) projected
  line L54 (28, -2.5) -> (28, -25.2604) projected
  line L55 (28, -24.35) -> (28, -25.85)
  line L56 (14.7, -40.85) -> (14.7, -28.85)
  line L57 (28, -25.85) -> (40, -25.85)
  line L58 (28, -24.35) -> (40, -24.35)
  line L59 (14.7, -40.85) -> (16.2, -40.85)
  line L60 (14.7, -28.85) -> (16.2, -28.85)
  line L61 (40, -24.35) -> (40, -25.85)
  line L62 (16.2, 40.85) -> (16.2, 28.85)
  line L63 (28, 24.35) -> (28, 25.85)
  line L64 (14.7, 40.85) -> (14.7, 28.85)
  line L65 (28, 25.85) -> (40, 25.85)
  line L66 (28, 24.35) -> (40, 24.35)
  line L67 (14.7, 40.85) -> (16.2, 40.85)
  line L68 (14.7, 28.85) -> (16.2, 28.85)
  line L69 (40, 24.35) -> (40, 25.85)
  line L70 (-16.2, -40.85) -> (-16.2, -28.85)
  line L71 (-28, -24.35) -> (-28, -25.85)
  line L72 (-14.7, -40.85) -> (-14.7, -28.85)
  line L73 (-28, -25.85) -> (-40, -25.85)
  line L74 (-28, -24.35) -> (-40, -24.35)
  line L75 (-14.7, -40.85) -> (-16.2, -40.85)
  line L76 (-14.7, -28.85) -> (-16.2, -28.85)
  line L77 (-40, -24.35) -> (-40, -25.85)
  line L78 (-28, 24.35) -> (-40, 24.35)
  line L79 (-28, 24.35) -> (-28, 25.85)
  line L80 (-40, 24.35) -> (-40, 25.85)
  line L81 (-28, 25.85) -> (-40, 25.85)
  line L82 (-14.7, 40.85) -> (-14.7, 28.85)
  line L83 (-14.7, 28.85) -> (-16.2, 28.85)
  line L84 (-16.2, 40.85) -> (-16.2, 28.85)
  line L85 (-14.7, 40.85) -> (-16.2, 40.85)
  point P0 (0, 0)
  point P1 (28, 25.2604)
  point P2 (-28, -25.2604)
  point P3 (-28, 25.2604)
  point P4 (16.2, -40.85)
  point P5 (-16.2, -40.85)
  point P6 (-14.7, -40.85)
  dimension "d54" = 7.3
  dimension "d55" = 1.5
  dimension "d67" = 1.5
  dimension "d68" = 23.8
  dimension "d69" = 15
  dimension "d70" = 1.5
  constraints: 160 end point, 63 symmetric about line, 5 point on line, 2 collinear, 2 horizontal, 1 coincident, 1 parallel, 1 perpendicular, 18 other
  measures "d54" distance between parallel lines of L3 L6
  measures "d55" distance between parallel lines of L6 L8
  measures "d67" distance between parallel lines of L57 L58
  measures "d68" distance between parallel lines of L50 L51
  measures "d69" distance between parallel lines of L57 L52
  measures "d70" distance between parallel lines of L56 L50
extrude "Ex-PlateMount1" cut sketch "S-PlateMount" along normal blind 2 from surface at -3 contours A0 | L2 L3 L4 L5 L6 L7 | L19 L18 L17 L16 L15 L14 | L31 L30 L29 L28 L27 L26 | L39 L42 L45 L47 L44 L40
extrude "Ex-PlateMount2" add sketch "S-PlateMount" along normal blind 1 from surface at 0 contours L52 L56 L53 L50 | L52 L70 L76 L72 | L57 L55 L54 L58 L51 | L66 L63 L65 L51 | L62 L68 L64 L67 | L71 L73 L77 L74 | L78 L80 L81 L79 | L82 L83 L84 L85
chamfer "Fase1" distance 1 angle 45 1 edges at (-3, 0, -3)
equation "\"d10\" = d8"
equation "\"d11\" = d4"
equation "\"d47\" = d49"
equation "\"d48\" = 2 * d49"
